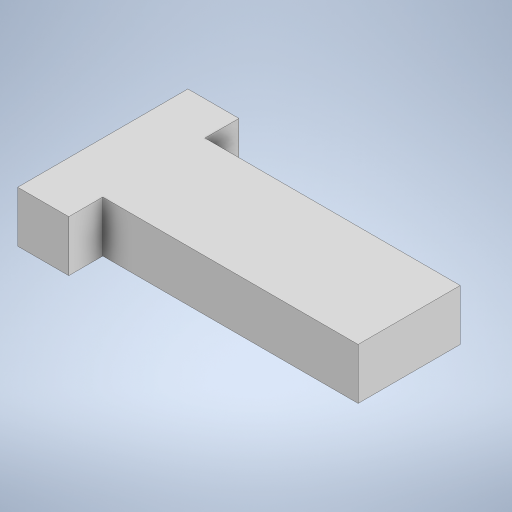
# Autodesk Inventor part: 插銷B
Saved by Autodesk Inventor 2024 (Build 280153000, 153)
## iProperties
Created: 2024-04-14
Part Number: 插銷B
Material: 一般
Document SubType Name: Modeling
Designer: USER
Density: 1 g/cm^3
Appearance: 預設
Author: USER
Autodesk Inventor part; units mm, degrees
ref_plane "YZ Plane" through (0, 0, 0) normal (1, 0, 0) x (0, 1, 0)
ref_plane "XZ Plane" through (0, 0, 0) normal (0, 1, 0) x (-1, 0, 0)
ref_plane "XY Plane" through (0, 0, 0) normal (0, 0, 1) x (1, 0, 0)
sketch "草圖1" plane through (0, 0, 0) normal (0, 1, 0) x (-1, 0, 0)
  line L0 (0, 3) -> (15, 3)
  line L1 (15, 3) -> (15, -3)
  line L2 (15, -3) -> (0, -3)
  line L3 (0, -3) -> (0, 3)
  line L4 (18, 5) -> (15, 5)
  line L5 (15, 5) -> (15, -5)
  line L6 (15, -5) -> (18, -5)
  line L7 (18, -5) -> (18, 5)
  point P0 (0, 0)
  point P1 (0, 0)
  point P2 (15, 0)
  dimension "d0" = 6
  dimension "d1" = 15
  dimension "d2" = 3
  dimension "d3" = 10
  constraints: 16 end point, 4 parallel, 3 midpoint, 2 horizontal, 2 perpendicular, 1 coincident
  measures "d0" distance of L2.end L0.start
  measures "d1" distance of L1.end L2.end
  measures "d2" distance of L5.end L6.end
  measures "d3" distance of L6.end L4.start
extrude "擠出1" add sketch "草圖1" along normal blind 3
